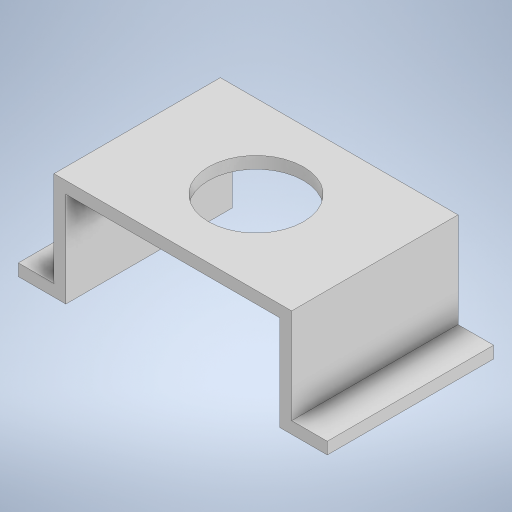
# Autodesk Inventor part: bunny offset
Saved by Autodesk Inventor 2024.2 (Build 282272000, 272)
## iProperties
Created: 2025-12-17
Part Number: bunny offset
Material: Generic
Document SubType Name: Modeling
Designer: David Toler II
Density: 1 g/cm^3
Appearance: Default
Author: David Toler II
Autodesk Inventor part; units mm, degrees
ref_plane "YZ Plane" through (0, 0, 0) normal (1, 0, 0) x (0, 1, 0)
ref_plane "XZ Plane" through (0, 0, 0) normal (0, 1, 0) x (-1, 0, 0)
ref_plane "XY Plane" through (0, 0, 0) normal (0, 0, 1) x (1, 0, 0)
sketch "Sketch1" plane through (0, 0, 0) normal (0, 0, 1) x (1, 0, 0)
  line L0 (-41.275, 0) -> (41.275, 0)
  line L1 (41.275, 0) -> (41.275, 28.575)
  line L2 (41.275, 28.575) -> (-41.275, 28.575)
  line L3 (-41.275, 28.575) -> (-41.275, 0)
  line L4 (-28.575, 28.575) -> (-28.575, 0)
  line L5 (28.575, 28.575) -> (28.575, 0)
  line L6 (-41.275, 25.4) -> (41.275, 25.4)
  line L7 (-31.75, 28.575) -> (-31.75, 0)
  line L8 (31.75, 28.575) -> (31.75, 0)
  line L9 (-41.275, 3.175) -> (41.275, 3.175)
  point P0 (0, 0)
  point P1 (0, 0)
  point P2 (-31.75, 3.175)
  point P3 (-28.575, 25.4)
  point P4 (28.575, 25.4)
  point P5 (31.75, 3.175)
  dimension "d0" = 28.575
  dimension "d1" = 12.7
  dimension "d2" = 12.7
  dimension "d3" = 57.15
  dimension "d4" = 3.175
  dimension "d5" = 3.175
  dimension "d6" = 3.175
  dimension "d7" = 3.175
  constraints: 20 end point, 12 point on line, 7 perpendicular, 2 parallel, 1 coincident, 1 horizontal, 1 midpoint
  measures "d0" distance between parallel lines of L0 L2
  measures "d1" distance between parallel lines of L4 L3
  measures "d2" distance between parallel lines of L1 L5
  measures "d3" distance between parallel lines of L5 L4
  measures "d4" distance between parallel lines of L2 L6
  measures "d5" distance between parallel lines of L4 L7
  measures "d6" distance between parallel lines of L5 L8
  measures "d7" distance between parallel lines of L0 L9
extrude "Extrusion1" add sketch "Sketch1" along normal blind 44.45 contours L3 L9 L7 L0 | L7 L9 L4 L0 | L7 L6 L4 L9 | L5 L9 L8 L0 | L7 L2 L4 L6 | L8 L9 L1 L0 | L5 L6 L8 L9 | L4 L2 L5 L6 | L5 L2 L8 L6
sketch "Sketch2" plane through (-31.75, 28.575, 0) normal (0, 1, 0) x (1, 0, 0)
  line L0 (63.5, 0) -> (0, 0) projected
  line L1 (0, 0) -> (0, -44.45) projected
  line L2 (63.5, -44.45) -> (0, -44.45) projected
  line L3 (63.5, 0) -> (63.5, -44.45) projected
  line L4 (31.75, 0) -> (31.75, -44.45)
  line L5 (0, -22.225) -> (63.5, -22.225)
  circle A0 centre (31.75, -22.225) radius 12.7
  dimension "d10" = 25.4
  constraints: 4 end point, 4 midpoint, 1 centre point
  measures "d10" diameter of A0
extrude "Extrusion2" cut sketch "Sketch2" against normal through all contours A0 L5 L4 | L4 L5 A0 | A0 L4 L5 | L4 A0 L5
body "Solid1"
